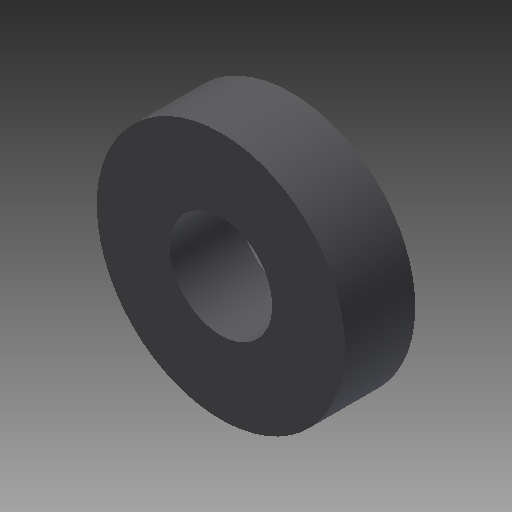
# Autodesk Inventor part: 0.750.212-rod_part0
Saved by Autodesk Inventor 2017 (Build 210142000, 142)
## iProperties
Category: PARTsolutions
Company: BIMBA
Created: 2017-01-25
Part Number: 0.750.212-rod_part0
Catalog Web Link: www.cadenas.de
Description: FO1-Rod Part-Bimba FLAT-1
Vendor: BIMBA
Document SubType Name: Modeling
Designer: psAdmin
Manufacturer: BIMBA
Mass: 1.27258 g
Surface Area: 9.28126 cm^2
Volume: 1.27258 cm^3
Density: 1 g/cm^3
Material: Generic
Appearance: PSOLRGB-180-180-180
PSOL_IDENT_0: {$CADENAS_DATA\23d-libs\bimba\bimba\bimba_imperial\bimba_full_line\flat_cylinders\fo1\fo1_rod_part.p
PSOL_IDENT_1: rj},191 {VTYP=3D},{NB=0.750.212-rod_part0},{LINA=0.750.212-rod_part0},{NN=FO1-Rod Part},{DATE=01.12.
PSOL_IDENT_2: 2016 06:16:11},{GEOMDATE=08.09.2015 08:56:00},{VERSION=},{LINEID=20},{LINESUBID=-1},{WBVAR=L,BCD}  {
PSOL_IDENT_3: NB=0.750.212-rod_part0},{LINA=0.750.212-rod_part0},{KT=DUMMY},{PN=0.750.212-rod_part0},{BORE=0.75000
PSOL_IDENT_4: 000},{L=0.212},{TDIN=0.75000000},{F=0.31000000},{BCD=0},{A=1.500}
NN: FO1-Rod Part
NT: Bimba FLAT-1
NB: 0.750.212-rod_part0
NBSYN: $PN.
LINA: 0.750.212-rod_part0
PN: 0.750.212-rod_part0
BORE: 0.75000000
L: 0.212
TDIN: 0.75000000
F: 0.31000000
BCD: 0
A: 1.500
SUPPLIER: BIMBA
ARTICLENO: 0.750.212-rod_part0
BOMINFO: 0.750.212-rod_part0
CREATOR: CADENAS GmbH
Title: 0.750.212-rod_part0
Author: Cadenas PARTsolutions
Comments: Bimba FLAT-1
Autodesk Inventor part; units mm, degrees
sketch "Sketch_1" plane through (0, 0, 0) normal (1, 0, 0) x (0, 1, 0)
  line L0 (0, -5.3848) -> (0, 0)
  line L1 (3.937, 0) -> (3.937, -5.3848)
  line L2 (3.937, -5.3848) -> (9.525, -5.3848)
  line L3 (9.525, -5.3848) -> (9.525, 0)
  line L4 (9.525, 0) -> (3.937, 0)
  constraints: 10 end point
revolve "Revolution1" add sketch "Sketch_1" angle 360 about axis through (0, 0, -5.3848) along (0, 0, -1)
ref_plane "part_to_rod_XY" through (0, 0, 0) normal (0, 0, 1) x (1, 0, 0)
ref_plane "part_to_rod_YZ" through (0, 0, 0) normal (1, 0, 0) x (0, 1, 0)
ref_plane "part_to_rod_ZX" through (0, 0, 0) normal (0, 1, 0) x (0, 0, 1)
body "Solid1"
